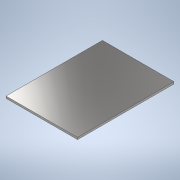
# Autodesk Inventor part: plate
Saved by Autodesk Inventor 2020 (Build 240168000, 168)
## iProperties
Created: 2020-07-26
Part Number: plate
Material: Stainless Steel
Document SubType Name: Modeling
Designer: Aarya
Density: 8 g/cm^3
Appearance: Semi-Polished
Author: Aarya
Autodesk Inventor part; units mm, degrees
ref_plane "YZ Plane" through (0, 0, 0) normal (1, 0, 0) x (0, 1, 0)
ref_plane "XZ Plane" through (0, 0, 0) normal (0, 1, 0) x (-1, 0, 0)
ref_plane "XY Plane" through (0, 0, 0) normal (0, 0, 1) x (1, 0, 0)
sketch "Sketch1" plane through (0, 0, 0) normal (0, 1, 0) x (-1, 0, 0)
  line L0 (36.1017, 48.6657) -> (-36.1017, 48.6657)
  line L1 (-36.1017, 48.6657) -> (-36.1017, -48.6657)
  line L2 (-36.1017, -48.6657) -> (36.1017, -48.6657)
  line L3 (36.1017, -48.6657) -> (36.1017, 48.6657)
  line L4 (36.1017, 48.6657) -> (-36.1017, -48.6657) construction
  line L5 (-36.1017, 48.6657) -> (36.1017, -48.6657) construction
  point P0 (0, 0)
  constraints: 12 end point, 2 midpoint, 2 parallel, 1 horizontal, 1 perpendicular
extrude "Extrusion1" add sketch "Sketch1" along normal blind 2
body "Solid1"
